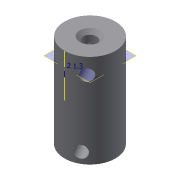
# Autodesk Inventor part: 00_Motorcoupling_5mm_M3
Saved by Autodesk Inventor 2022 (Build 260153000, 153)
## iProperties
Created: 2021-04-26
Part Number: 00_Motorcoupling_5mm_M3
Material: Generic
Document SubType Name: Modeling
Designer: diederichbenedict
Density: 1 g/cm^3
Appearance: Default
Mass: 1.15069 g
Surface Area: 11.4691 cm^2
Volume: 1.15069 cm^3
Author: diederichbenedict
Autodesk Inventor part; units mm, degrees
ref_plane "YZ Plane" through (0, 0, 0) normal (1, 0, 0) x (0, 1, 0)
ref_plane "XZ Plane" through (0, 0, 0) normal (0, 1, 0) x (-1, 0, 0)
ref_plane "XY Plane" through (0, 0, 0) normal (0, 0, 1) x (1, 0, 0)
sketch "Sketch1" plane through (0, 0, 0) normal (0, 1, 0) x (-1, 0, 0)
  circle A0 centre (0, 0) radius 6
  line L0 (0, -8.6) -> (0, 9.6) construction
  circle A1 centre (0, 0) radius 1.4
  dimension "d0" = 12
  dimension "d42" = 2.8
  constraints: 2 centre point, 1 coincident
  measures "d0" diameter of A0
  measures "d42" diameter of A1
extrude "Extrusion1" add sketch "Sketch1" along normal blind 10
sketch "Sketch2" plane through (0, 0, 0) normal (0, -1, 0) x (1, 0, 0)
  circle A0 centre (0, 0) radius 1.45
  arc A1 (1.28938, -2.2) -> (-1.28938, -2.2) centre (0, 0) ccw
  line L0 (-1.28938, -2.2) -> (1.28938, -2.2)
  circle A2 centre (0, 0) radius 6
  arc A3 (-1.28938, -2.2) -> (1.28938, -2.2) centre (0, 0) ccw
  dimension "d4" = 5.1
  dimension "d5" = 2.2
  constraints: 5 point on circle, 2 centre point, 2 coincident, 2 end point, 1 horizontal
  measures "d4" diameter of A1
  measures "d5" distance from line of L0 point (0, 0)
extrude "Extrusion2" add sketch "Sketch2" along normal blind 12 contours A2
ref_plane "Work Plane1" through (0, 6, 0) normal (0, -1, 0) x (1, 0, 0)
sketch "Sketch5" plane through (0, 0, 0) normal (1, 0, 0) x (0, 1, 0)
  line L0 (0, 6) -> (10, 6)
  line L1 (4.694209, 6) -> (5.994209, 6)
  line L2 (5.994209, 6) -> (5.994209, 4)
  line L3 (5.994209, 4) -> (4.694209, 4)
  line L4 (4.694209, 4) -> (4.694209, 6)
  point P0 (0, 0)
  dimension "d17" = 1.3
  dimension "d18" = 2
  constraints: 8 end point, 2 parallel, 1 horizontal, 1 perpendicular, 1 point on line
  measures "d17" distance of L2.end L3.end
  measures "d18" distance of L1.end L2.end
sketch "Sketch6" plane through (0, 0, 0) normal (1, 0, 0) x (0, 1, 0)
  circle A0 centre (6.266092, 1) radius 1.4
  line L0 (-12, -6) -> (10, -6)
  circle A1 centre (-9.523155, 0) radius 1.4
  point P0 (0, 0)
  dimension "d43" = 2.8
  dimension "d44" = 7
  dimension "d56" = 2.8
  constraints: 2 centre point
  measures "d43" diameter of A0
  measures "d44" distance from line of A0.centre L0
  measures "d56" diameter of A1
extrude "Extrusion5" cut sketch "Sketch6" against normal blind 10
pattern_circular "Circular Pattern3" count 3 over 360 about axis through (0, 0, 0) along (0, 1, 0) of "Extrusion5"
chamfer "Chamfer4" distance 1 angle 45 2 edges at (1.4, 10, 0) (0, -12, 2.55)
sketch "Sketch7" plane through (0, 10, 0) normal (0, 1, 0) x (1, 0, 0)
  circle A0 centre (0, 0) radius 1.4 projected
  circle A1 centre (0, 0) radius 1.6
  dimension "d53" = 3.2
  constraints: 1 centre point, 1 coincident
  measures "d53" diameter of A1
sketch "Sketch7 outline for Extrusion6" plane through (0, 10, 0) normal (0, 1, 0) x (1, 0, 0)
  circle A0 centre (0, 0) radius 1.6
extrude "Extrusion6" cut sketch "Sketch7 outline for Extrusion6" against normal blind 10 draft -2
body "Solid1"
